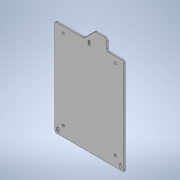
# Autodesk Inventor part: TBD_Box_Fix
Saved by Autodesk Inventor 2022 (Build 260153000, 153)
## iProperties
Created: 2020-10-24
Part Number: TBD_Box_Fix
Material: Generic
Document SubType Name: Modeling
Designer: lgnds
Density: 1 g/cm^3
Appearance: Default
Sheet Metal Rule: Default_mm
Author: lgnds
Autodesk Inventor part; units mm, degrees
ref_plane "YZ Plane" through (0, 0, 0) normal (1, 0, 0) x (0, 1, 0)
ref_plane "XZ Plane" through (0, 0, 0) normal (0, 1, 0) x (-1, 0, 0)
ref_plane "XY Plane" through (0, 0, 0) normal (0, 0, 1) x (1, 0, 0)
sketch "Sketch1" plane through (0, 0, 0) normal (0, 0, 1) x (1, 0, 0)
  line L0 (-82.5, -114.5) -> (82.5, -114.5)
  line L1 (82.5, -114.5) -> (82.5, 114.5)
  line L2 (82.5, 114.5) -> (-82.5, 114.5)
  line L3 (-82.5, 114.5) -> (-82.5, -114.5)
  line L4 (-82.5, -114.5) -> (82.5, 114.5) construction
  line L5 (82.5, -114.5) -> (-82.5, 114.5) construction
  circle A0 centre (61.5, 99.5) radius 2.5
  line L6 (-147.2223, 0) -> (154.3177, 0) construction
  line L7 (-104.1452, 5) -> (111.2405, 5) construction
  circle A1 centre (61.5, -89.5) radius 2.5
  line L8 (0, 191.5) -> (0, -165.5) construction
  circle A2 centre (-61.5, 99.5) radius 2.5
  circle A3 centre (-61.5, -89.5) radius 2.5
  line L9 (41.5, 114.5) -> (41.5, 140.5)
  line L10 (41.5, 140.5) -> (13.216, 140.5)
  line L11 (13.216, 140.5) -> (-12.784, 114.5)
  point P0 (0, 0)
  dimension "d0" = 229
  dimension "d1" = 165
  dimension "d3" = 5
  dimension "d5" = 189
  dimension "d6" = 25
  dimension "d9" = 61.5
  dimension "d31" = 41
  dimension "d32" = 26
  dimension "d33" = 135
  dimension "d34" = 28.284
  measures "d0" distance of L2.end L0.start
  measures "d1" distance of L1.end L2.end
  measures "d3" diameter of A0
  measures "d5" distance of A1.centre A0.centre
  measures "d6" distance from line of L0 A1.centre
  measures "d9" horizontal distance of point (0, 0) A0.centre
  measures "d31" distance between parallel lines of L1 L9
  measures "d32" distance of L9.start L9.end
  measures "d33" angle of L10 L11
  measures "d34" distance from line of L10.end L9
extrude "Plate1" add sketch "Sketch1" along normal blind 3
fillet "Fillet1" radius 5 4 edges at (-82.5, 114.5, 1.5) (82.5, 114.5, 1.5) (82.5, -114.5, 1.5) (-82.5, -114.5, 1.5)
sketch "Sketch2" plane through (0, 0, 3) normal (0, 0, 1) x (1, 0, 0)
  line L0 (-74.3, -107) -> (-74.3, -102) construction
  line L1 (-76.95, -107) -> (-76.95, -102)
  line L2 (-71.65, -102) -> (-71.65, -107)
  arc A0 (-76.95, -107) -> (-71.65, -107) centre (-74.3, -107) ccw
  arc A1 (-71.65, -102) -> (-76.95, -102) centre (-74.3, -102) ccw
  line L3 (-103.0799, -19.5) -> (98.9164, -19.5) construction
  line L4 (0, 191.5) -> (0, -165.5) construction
  line L5 (-82.5, -109.5) -> (-82.5, 109.5) construction
  line L6 (74.3, -107) -> (74.3, -102) construction
  line L7 (76.95, -107) -> (76.95, -102)
  line L8 (71.65, -102) -> (71.65, -107)
  arc A2 (71.65, -107) -> (76.95, -107) centre (74.3, -107) ccw
  arc A3 (76.95, -102) -> (71.65, -102) centre (74.3, -102) ccw
  line L9 (77.5, -114.5) -> (-77.5, -114.5) projected
  line L10 (0, 113) -> (0, 108) construction
  line L11 (-2.65, 113) -> (-2.65, 108)
  line L12 (2.65, 108) -> (2.65, 113)
  arc A4 (2.65, 113) -> (-2.65, 113) centre (0, 113) ccw
  arc A5 (-2.65, 108) -> (2.65, 108) centre (0, 108) ccw
  line L13 (-77.5, 114.5) -> (77.5, 114.5) projected
  point P0 (0, 0)
  point P1 (-74.3, -104.5)
  point P2 (74.3, -104.5)
  point P3 (82.5, -109.5)
  point P4 (0, 110.5)
  dimension "d12" = 85
  dimension "d14" = 5
  dimension "d15" = 2.65
  dimension "d18" = 10
  dimension "d22" = 148.6
  dimension "d23" = 5
  dimension "d24" = 2.65
  dimension "d26" = 225
  constraints: 26 end point, 12 point on circle, 8 symmetric about line, 8 tangent, 6 centre point, 2 midpoint, 2 parallel, 2 point on line, 1 horizontal, 1 vertical, 2 other
  measures "d12" distance from line of L3 point (-74.3, -104.5)
  measures "d14" distance of L2.start L2.end
  measures "d15" radius of A1
  measures "d18" distance from line of L9 point (-74.3, -104.5)
  measures "d22" distance of point (74.3, -104.5) point (-74.3, -104.5)
  measures "d23" distance of L12.start L12.end
  measures "d24" radius of A4
  measures "d26" distance from line of L9 point (0, 110.5)
extrude "Cut1" cut sketch "Sketch2" against normal blind 3
fillet "Fillet2" radius 5 4 edges at (41.5, 114.5, 1.5) (41.5, 140.5, 1.5) (13.216, 140.5, 1.5) (-12.784, 114.5, 1.5)
chamfer "Chamfer1" distance 0.75 angle 45 14 edges at (0, -114.5, 3) (-81.0355, -113.0355, 3) (-82.5, 0, 3) (-81.0355, 113.0355, 3) (-46.1775, 114.5, 3) (13.3737, 140.1194, 3) (40.0355, 139.0355, 3) (0.216, 127.5, 3) (25.8935, 140.5, 3) (41.5, 127.5, 3) (62, 114.5, 3) (81.0355, 113.0355, 3) (82.5, 0, 3) (81.0355, -113.0355, 3)
sketch "Sketch4" plane through (0, 0, 3) normal (0, 0, 1) x (1, 0, 0)
  circle A0 centre (85, -108.7631) radius 2
  line L0 (82.5, -109.5) -> (82.5, 109.5) projected
  point P0 (0, 0)
  dimension "d35" = 2.5
  dimension "d36" = 4
  constraints: 1 centre point
  measures "d35" distance from line of L0 A0.centre
  measures "d36" diameter of A0
equation "\"d18\" = d13"
equation "\"d3\" = d2"
equation "\"d15\" = d24"
equation "\"d23\" = d14"
equation "\"d16\" = Thickness"
equation "\"d10\" = Thickness"
equation "\"BendRadius\" = Thickness"
equation "\"BendReliefWidth\" = Thickness"
equation "\"BendReliefDepth\" = 0.5 * Thickness"
equation "\"CornerReliefSize\" = 4 * Thickness"
equation "\"MinimumRemnant\" = 2 * Thickness"
equation "\"TransitionRadius\" = BendRadius"
equation "\"JacobiRadiusSize\" = BendRadius"
equation "\"GapSize\" = Thickness"
equation "\"d2\" = 5"
equation "\"Thickness\" = 3"
equation "\"d13\" = 10"
body "Solid1"
